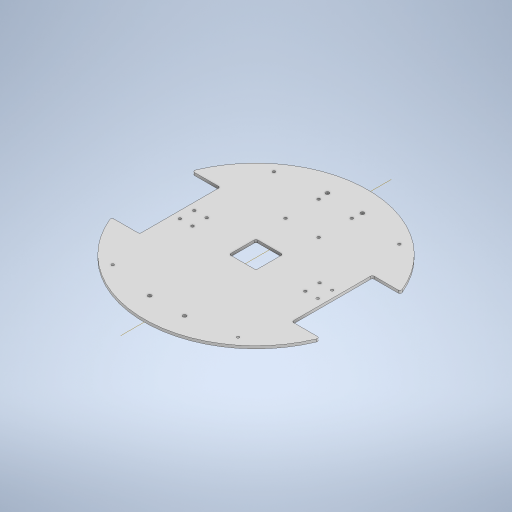
# Autodesk Inventor part: Part1
Saved by Autodesk Inventor 2023.3 (Build 273359000, 359)
## iProperties
Created: 2023-08-25
Part Number: Part1
Material: Generic
Document SubType Name: Modeling
Designer: husse
Density: 1 g/cm^3
Appearance: Default
Author: husse
Autodesk Inventor part; units mm, degrees
ref_plane "YZ Plane" through (0, 0, 0) normal (1, 0, 0) x (0, 1, 0)
ref_plane "XZ Plane" through (0, 0, 0) normal (0, 1, 0) x (-1, 0, 0)
ref_plane "XY Plane" through (0, 0, 0) normal (0, 0, 1) x (1, 0, 0)
sketch "Sketch1" plane through (0, 0, 0) normal (0, 1, 0) x (-1, 0, 0)
  line L0 (-85, 43) -> (-85, -43)
  line L1 (85, -43) -> (85, 43)
  arc A0 (-115.5144, -47.7642) -> (115.5144, -47.7642) centre (0, 0) ccw
  arc A1 (115.5144, 47.7642) -> (-115.5144, 47.7642) centre (0, 0) ccw
  line L2 (113.6662, 45) -> (87, 45)
  line L3 (-87, 45) -> (-113.6662, 45)
  line L4 (87, -45) -> (113.6662, -45)
  line L5 (-113.6662, -45) -> (-87, -45)
  circle A2 centre (63, -8) radius 1.5
  circle A3 centre (63, 8) radius 1.5
  circle A4 centre (77, 8) radius 1.5
  circle A5 centre (77, -8) radius 1.5
  circle A6 centre (-63, -8) radius 1.5
  circle A7 centre (-63, 8) radius 1.5
  circle A8 centre (-77, 8) radius 1.5
  circle A9 centre (-77, -8) radius 1.5
  circle A10 centre (70, -90) radius 1.5
  circle A11 centre (-70, -90) radius 1.5
  circle A12 centre (-70, 90) radius 1.5
  circle A13 centre (70, 90) radius 1.5
  line L6 (13, 15) -> (-13, 15)
  line L7 (-15, 13) -> (-15, -13)
  line L8 (-13, -15) -> (13, -15)
  line L9 (15, -13) -> (15, 13)
  circle A14 centre (-18.5, -51.5) radius 1.5
  circle A15 centre (-18.5, -88.5) radius 1.5
  circle A16 centre (18.5, -88.5) radius 1.5
  circle A17 centre (18.5, -51.5) radius 1.5
  arc A18 (115.5144, -47.7642) -> (113.6662, -45) centre (113.6662, -47) ccw
  arc A19 (85, -43) -> (87, -45) centre (87, -43) ccw
  arc A20 (87, 45) -> (85, 43) centre (87, 43) ccw
  arc A21 (113.6662, 45) -> (115.5144, 47.7642) centre (113.6662, 47) ccw
  arc A22 (-115.5144, 47.7642) -> (-113.6662, 45) centre (-113.6662, 47) ccw
  arc A23 (-85, 43) -> (-87, 45) centre (-87, 43) ccw
  arc A24 (-87, -45) -> (-85, -43) centre (-87, -43) ccw
  arc A25 (-113.6662, -45) -> (-115.5144, -47.7642) centre (-113.6662, -47) ccw
  arc A26 (-15, -13) -> (-13, -15) centre (-13, -13) ccw
  arc A27 (-13, 15) -> (-15, 13) centre (-13, 13) ccw
  arc A28 (15, 13) -> (13, 15) centre (13, 13) ccw
  arc A29 (13, -15) -> (15, -13) centre (13, -13) ccw
  circle A30 centre (-19.5, -99.2842) radius 2
  circle A31 centre (19.5, -99.2842) radius 2
  circle A32 centre (-19.5, 99.2842) radius 2
  circle A33 centre (19.5, 99.2842) radius 2
  point P0 (116.619, -45)
  point P1 (116.619, 45)
  point P2 (-116.619, 45)
  point P3 (-116.619, -45)
  point P4 (85, 0)
  constraints: 34 centre point, 32 point on circle, 20 end point, 8 horizontal, 8 tangent, 5 parallel, 4 point on line, 4 vertical, 1 coincident, 1 midpoint, 76 other
extrude "Extrusion2" add sketch "Sketch1" along normal blind 3
body "Solid2"
